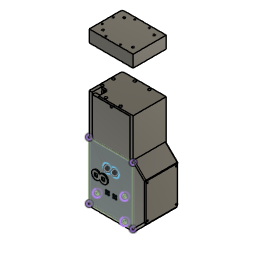
ExternalCardReaderHousingV3 v20 (Autodesk Fusion 360 design; units mm, degrees)
Autodesk Fusion 360 part; units mm, degrees
note: some values were not read from the file. Set by a fixed rule: which face or edge a step refers to.
(part 1 of 2)
sketch "ReaderBodyHalf" plane through (0, 0, 0) normal (0, 0, 1) x (1, 0, 0)
  line L0 (0, 0) -> (102, 0)
  line L1 (102, 0) -> (102, 38.5)
  line L2 (102, 38.5) -> (0, 38.5)
  line L3 (0, 38.5) -> (0, 0)
  line L4 (7, 7) -> (95, 7)
  line L5 (95, 7) -> (95, 38.5)
  line L6 (7, 38.5) -> (7, 7)
  circle A0 centre (90.5, 11.5) radius 1.75
  circle A1 centre (90.5, 11.5) radius 5.75
  circle A2 centre (11.5, 11.5) radius 1.75
  circle A3 centre (11.5, 11.5) radius 5.75
  line L7 (90.5, 17.25) -> (95, 17.25)
  line L8 (90.5, 11.5) -> (84.75, 11.5)
  line L9 (84.75, 7) -> (84.75, 11.5)
  line L10 (11.5, 17.25) -> (7, 17.25)
  line L11 (17.25, 11.5) -> (17.25, 7)
  line L12 (95, 17.25) -> (102, 17.25)
  line L13 (95, 7) -> (102, 7)
  circle A4 centre (34, 5) radius 2.35
  circle A5 centre (34, 5) radius 5
  circle A6 centre (34, 5) radius 5
  circle A7 centre (34, 5) radius 2.35
  circle A8 centre (68, 5) radius 5
  circle A9 centre (68, 5) radius 2.35
  circle A10 centre (5, 25.6667) radius 5
  circle A11 centre (5, 25.6667) radius 2.35
  circle A12 centre (90.5, 11.5) radius 0.7071
  circle A13 centre (68, 5) radius 1.75
  circle A14 centre (34, 5) radius 1.75
  circle A15 centre (5, 25.6667) radius 1.75
  circle A16 centre (5, 25.6667) radius 3
  circle A17 centre (34, 5) radius 3
  circle A18 centre (68, 5) radius 3
  line L14 (71, 5) -> (71, 7)
  line L15 (65, 5) -> (65, 7)
  line L16 (37, 5) -> (37, 7)
  line L17 (31, 5) -> (31, 7)
  line L18 (5, 22.6667) -> (7, 22.6667)
  line L19 (5, 28.6667) -> (7, 28.6667)
  dimension "d1" = 102
  dimension "d9" = 7
  dimension "d10" = 7
  dimension "d21" = 11.5
  dimension "d23" = 11.5
  dimension "d24" = 3.5
  dimension "d25" = 3.5
  dimension "d29" = 11.5
  dimension "d30" = 11.5
  dimension "d31" = 11.5
  dimension "d32" = 11.5
  dimension "d33" = 11.5
  dimension "d34" = 11.5
  dimension "d35" = 11.5
  dimension "d36" = 11.5
  dimension "d166" = 4.7
  dimension "d167" = 10
  dimension "d168" = 34
  dimension "d169" = 4.7
  dimension "d170" = 10
  dimension "d175" = 10
  dimension "d176" = 4.7
  dimension "d178" = 34
  dimension "d179" = 34
  dimension "d184" = 4.7
  dimension "d185" = 10
  dimension "d303" = 25.6667
  dimension "d340" = 38.5
  dimension "d392" = 3.5
  dimension "d393" = 3.5
  dimension "d394" = 3.5
  dimension "d470" = 6
  dimension "d471" = 6
  dimension "d472" = 6
  constraint horizontal L0
  constraint vertical L1
  constraint horizontal L2
  constraint vertical L3
  constraint coincident L0.start L3.end
  constraint horizontal L4
  constraint vertical L5
  constraint vertical L6
  constraint coincident A1 L7.start
  constraint tangent A1 L7
  constraint coincident L5 L7.end
  constraint perpendicular L5 L7
  constraint coincident A0.centre A1.centre
  constraint coincident A1 L8.end
  constraint parallel L4 L8
  constraint coincident L4 L9.start
  constraint tangent A1 L9
  constraint coincident A3 L10.start
  constraint coincident L6 L10.end
  constraint tangent A3 L10
  constraint perpendicular L6 L10
  constraint coincident A3 L11.start
  constraint coincident L4 L11.end
  constraint tangent A3 L11
  constraint perpendicular L4 L11
  constraint coincident L1 L12.end
  constraint perpendicular L1 L12
  constraint coincident L1 L13.end
  constraint perpendicular L1 L13
  constraint concentric A4 A5
  constraint concentric A6 A7
  constraint concentric A10 A11
  constraint coincident L2 L5.end
  constraint coincident L2 L6.start
  constraint concentric A1 A12
  constraint concentric A9 A13
  constraint concentric A5 A14
  constraint concentric A10 A15
  constraint concentric A10 A16
  constraint concentric A14 A17
  constraint concentric A13 A18
  constraint coincident A18 L14.start
  constraint coincident L4 L14.end
  constraint tangent A18 L14
  constraint perpendicular L4 L14
  constraint coincident A18 L15.start
  constraint coincident L4 L15.end
  constraint tangent A18 L15
  constraint perpendicular L4 L15
  constraint coincident A17 L16.start
  constraint coincident L4 L16.end
  constraint tangent A17 L16
  constraint perpendicular L4 L16
  constraint coincident A17 L17.start
  constraint coincident L4 L17.end
  constraint tangent A17 L17
  constraint perpendicular L4 L17
  constraint coincident A16 L18.start
  constraint coincident L6 L18.end
  constraint tangent A16 L18
  constraint perpendicular L6 L18
  constraint coincident A16 L19.start
  constraint coincident L6 L19.end
  constraint tangent A16 L19
  constraint perpendicular L6 L19
  measures "d1" distance of L0.start L0.end
  measures "d9" distance of L3 L6
  measures "d10" distance of L0 L4
  measures "d21" diameter of A3
  measures "d23" diameter of A1
  measures "d24" diameter of A0
  measures "d25" diameter of A2
  measures "d29" distance of L0 A0.centre
  measures "d30" distance of L1 A0.centre
  measures "d31" distance of L0 A2.centre
  measures "d32" distance of L3 A2.centre
  measures "d33" distance of L3 A2.centre
  measures "d34" distance of L0 A2.centre
  measures "d35" distance of L0 A0.centre
  measures "d36" distance of L1 A0.centre
  measures "d166" diameter of A4
  measures "d167" diameter of A5
  measures "d168" distance of L3 A4.centre
  measures "d169" diameter of A7
  measures "d170" diameter of A6
  measures "d175" diameter of A8
  measures "d176" diameter of A9
  measures "d178" distance of L1 A8.centre
  measures "d179" distance of L1 A8.centre
  measures "d184" diameter of A11
  measures "d185" diameter of A10
  measures "d303" distance of L0 A10.centre
  measures "d340" distance of L0.start L2.end
  measures "d392" diameter of A13
  measures "d393" diameter of A14
  measures "d394" diameter of A15
  measures "d470" diameter of A16
  measures "d471" diameter of A17
  measures "d472" diameter of A18
extrude "Extrude1" add sketch "ReaderBodyHalf" along normal blind 134 contours L0 L3 L4 L6 A3 A5 A6 A10 | L0 L4 A5 A6 A8 | L4 A5 A6 A17 L16 L17 | L2 L3 L6 A10 | L6 A10 A16 L18 L19 | L0 L1 L4 A1 L13 A8 | L4 A8 A18 L14 L15 | L4 A17 L17 | L6 A16 L19 | L6 A16 L18 | L4 A18 L15 | L4 A3 | L4 A4 A7 A17 | L4 A17 L16 | L6 A11 A16 | L6 A3 | L4 A9 A18 | L4 A18 L14 | L4 A4 A7 | L6 A11 | L4 A1 | L4 A9 | A13 | A14 | A15 picked at (31.228, 4.8338) picked at (4.8372, 28.4387) picked at (65.228, 4.8338) picked at (32.7196, 6.7212) picked at (2.8543, 25.6667) picked at (66.7196, 6.7212) makes body 1
extrude "Extrude2" add sketch "ReaderBodyHalf" along normal blind 6 contours L4 A3 L11 | L6 A3 L10 | L1 L5 A1 L12 L13 | L4 L6 A3 | L4 L5 A1 | L4 A1 L9 | L4 L6 A3 | L5 A1 L7 | L4 L5 A1 | L5 A1 bodies 1
extrude "Extrude16" add sketch "ReaderBodyHalf" against normal blind 8 from surface at 134 contours L4 A5 A6 A17 | L6 A10 A16 | L4 A8 A18 | L4 A4 A7 A17 | L6 A11 A16 | L4 A9 A18 | L4 A4 A7 | L6 A11 | L4 A9 picked at (32.6487, 7.4264) picked at (7.4264, 27.018) picked at (66.6487, 7.4264) picked at (34, 7.1167) picked at (7.0503, 25.3511) picked at (68.0958, 7.167) bodies 1
revolve "Revolve4" add 1 faces at (68.353, 8.1961, 126) angle 90 about axis through (63.4174, 7, 126) along (-1, 0, 0) on bodies 1 bodies 1
revolve "Revolve5" add 1 faces at (32.9452, 8.3501, 126) angle 90 about axis through (29.4174, 7, 126) along (-1, 0, 0) on bodies 1 bodies 1
revolve "Revolve6" add 1 faces at (8.3577, 25.1904, 126) angle 90 about axis through (7, 30.2492, 126) along (0, 1, 0) on bodies 1 bodies 1
extrude "Extrude17" cut sketch "ReaderBodyHalf" against normal blind 4 from surface at 134 contours L4 A4 A7 | L4 A4 A7 | L6 A11 | L6 A11 | L4 A9 | L4 A9 | A13 | A14 | A15 bodies 1
sketch "TopInsertHole alighment" plane through (102, 0, 0) normal (1, 0, 0) x (0, 1, 0)
  line L0 (0, 0) -> (17.25, 0)
  line L1 (17.25, 6) -> (7, 6)
  line L2 (0, 0) -> (77, 0)
  line L3 (77, 0) -> (77, 109.8006)
  line L4 (77, 109.8006) -> (0, 109.8006)
  line L5 (0, 109.8006) -> (0, 0)
  circle A0 centre (72, 28) radius 5
  circle A1 centre (72, 28) radius 2.35
  circle A2 centre (72, 104.8006) radius 2.35
  circle A3 centre (72, 104.8006) radius 5
  circle A4 centre (5, 104.8006) radius 2.35
  circle A5 centre (5, 104.8006) radius 5
  circle A6 centre (5, 28) radius 2.35
  circle A7 centre (5, 28) radius 5
  line L6 (64, 97.8006) -> (13, 97.8006)
  line L7 (13, 97.8006) -> (13, 33.8006)
  line L8 (13, 33.8006) -> (64, 33.8006)
  line L9 (64, 33.8006) -> (64, 97.8006)
  circle A8 centre (59.5, 89.0506) radius 2.35
  circle A9 centre (59.5, 43.0506) radius 2.35
  circle A10 centre (59.5, 89.0506) radius 5
  circle A11 centre (59.5, 43.0506) radius 5
  circle A12 centre (72, 28) radius 1.75
  circle A13 centre (72, 104.8006) radius 1.75
  circle A14 centre (5, 28) radius 1.75
  circle A15 centre (5, 104.8006) radius 1.75
  line L10 (17.25, 0) -> (17.25, 6)
  line L11 (0, 134) -> (0, 0)
  line L12 (7, 6) -> (7, 134)
  line L13 (7, 134) -> (0, 134)
  circle A16 centre (17.5, 89.0506) radius 5
  circle A17 centre (17.5, 89.0506) radius 2.35
  circle A18 centre (17.5, 43.0506) radius 5
  circle A19 centre (17.5, 43.0506) radius 2.35
  line L14 (77, 0) -> (77, -7)
  line L15 (77, -7) -> (0, -7)
  line L16 (0, -7) -> (0, 0)
  dimension "d218" = 10
  dimension "d219" = 5
  dimension "d221" = 4.7
  dimension "d222" = 4.7
  dimension "d223" = 4.7
  dimension "d224" = 4.7
  dimension "d225" = 10
  dimension "d226" = 10
  dimension "d227" = 10
  dimension "d231" = 5
  dimension "d232" = 5
  dimension "d233" = 5
  dimension "d280" = 64
  dimension "d281" = 51
  dimension "d282" = 13
  dimension "d283" = 12
  dimension "d284" = 4.7
  dimension "d285" = 4.7
  dimension "d286" = 4.5
  dimension "d287" = 4.5
  dimension "d288" = 8.75
  dimension "d289" = 46
  dimension "d290" = 10
  dimension "d291" = 10
  dimension "d295" = 3.5
  dimension "d296" = 3.5
  dimension "d297" = 3.5
  dimension "d298" = 3.5
  dimension "d346" = 4.7
  dimension "d347" = 4.7
  dimension "d348" = 46
  dimension "d349" = 10
  dimension "d350" = 10
  dimension "d351" = 4.5
  dimension "d352" = 4.5
  dimension "d353" = 7
  dimension "d354" = 35
  dimension "d355" = 35
  dimension "d357" = 5
  dimension "d358" = 5
  dimension "d359" = 8.75
  dimension "d360" = 13
  constraint horizontal L2
  constraint vertical L3
  constraint horizontal L4
  constraint vertical L5
  constraint coincident L0.start L2.start
  constraint concentric A0 A1
  constraint concentric A2 A3
  constraint concentric A4 A5
  constraint concentric A6 A7
  constraint horizontal L6
  constraint vertical L7
  constraint horizontal L8
  constraint vertical L9
  constraint concentric A8 A10
  constraint concentric A9 A11
  constraint concentric A0 A12
  constraint concentric A3 A13
  constraint concentric A7 A14
  constraint concentric A5 A15
  constraint concentric A16 A17
  constraint concentric A18 A19
  constraint perpendicular L2 L14
  constraint perpendicular L14 L15
  constraint perpendicular L2 L16
  measures "d218" diameter of A0
  measures "d219" distance of L3 A0.centre
  measures "d221" diameter of A1
  measures "d222" diameter of A6
  measures "d223" diameter of A4
  measures "d224" diameter of A2
  measures "d225" diameter of A7
  measures "d226" diameter of A5
  measures "d227" diameter of A3
  measures "d231" distance of L5 A6.centre
  measures "d232" distance of L5 A4.centre
  measures "d233" distance of L3 A2.centre
  measures "d280" distance of L6.end L7.end
  measures "d281" distance of L6.start L6.end
  measures "d282" distance of L3 L9
  measures "d283" distance of L4 L6
  measures "d284" diameter of A8
  measures "d285" diameter of A9
  measures "d286" distance of L9 A8.centre
  measures "d287" distance of L9 A9.centre
  measures "d288" distance of L6 A8.centre
  measures "d289" distance of A8.centre A9.centre
  measures "d290" diameter of A10
  measures "d291" diameter of A11
  measures "d295" diameter of A12
  measures "d296" diameter of A13
  measures "d297" diameter of A14
  measures "d298" diameter of A15
  measures "d346" diameter of A17
  measures "d347" diameter of A19
  measures "d348" distance of A16.centre A18.centre
  measures "d349" diameter of A16
  measures "d350" diameter of A18
  measures "d351" distance of L7 A16.centre
  measures "d352" distance of L7 A18.centre
  measures "d353" distance of L2.end L14.end
  measures "d354" distance of A0.centre L15
  measures "d355" distance of A6.centre L15
  measures "d357" distance of L4 A2.centre
  measures "d358" distance of L4 A4.centre
  measures "d359" distance of L6 A16.centre
  measures "d360" distance of L5 L7
extrude "Extrude18" add sketch "TopInsertHole alighment" against normal blind 8 contours A6 A7 L12 | A4 A5 L12 | A6 A7 L12 | A4 A5 L12 | A6 L12 | A6 L12 | A4 L12 | A4 L12 | A14 | A15 bodies 1
extrude "Extrude19" cut sketch "TopInsertHole alighment" against normal blind 4 contours A6 L12 | A6 L12 | A4 L12 | A4 L12 | A14 | A15 bodies 1
extrude "Extrude29" cut sketch "TopInsertHole alighment" against normal blind 3 from surface at -4 contours A14 | A15 bodies 1
mirror "Mirror1" about plane through (7, 38.5, 0) normal (0, 1, 0) of bodies 1 makes body 2
sketch "PingulpMount" plane through (0, 0, 0) normal (0, 1, 0) x (1, 0, 0)
  line L0 (0, -1.75) -> (0, -22.5)
  circle A0 centre (18.5001, -30.5) radius 2.5
  circle A1 centre (82.5001, -5) radius 4.25
  line L1 (89.0001, 6) -> (89.0001, -68)
  line L2 (0.0001, -68) -> (0.0001, 6)
  circle A2 centre (18.5001, -30.5) radius 4.25
  circle A3 centre (82.5001, -56) radius 4.25
  circle A4 centre (82.5001, -5) radius 2.5
  line L3 (0.0001, 6) -> (89.0001, 6)
  circle A5 centre (82.5001, -56) radius 2.5
  line L4 (89.0001, -68) -> (0.0001, -68)
  point P0 (5, 0)
  dimension "d324" = 74
  dimension "d325" = 89
  dimension "d326" = 0.0001
  dimension "d327" = 5
  dimension "d328" = 5
  dimension "d329" = 5
  dimension "d330" = 6.5
  dimension "d331" = 11
  dimension "d332" = 6.5
  dimension "d333" = 51
  dimension "d334" = 36.5
  dimension "d335" = 70.5
  dimension "d336" = 8.5
  dimension "d337" = 8.5
  dimension "d338" = 8.5
  constraint horizontal L3
  constraint vertical L1
  constraint horizontal L4
  constraint vertical L2
  constraint concentric A0 A2
  constraint concentric A3 A5
  constraint concentric A1 A4
  measures "d324" distance of L2.end L2.start
  measures "d325" distance of L1.start L2.end
  measures "d326" distance of L0 L2
  measures "d327" diameter of A0
  measures "d328" diameter of A5
  measures "d329" diameter of A4
  measures "d330" distance of A1.centre L1
  measures "d331" distance of A1.centre L3
  measures "d332" distance of A3.centre L1
  measures "d333" distance of A3.centre A1.centre
  measures "d334" distance of A0.centre L3
  measures "d335" distance of A0.centre L1
  measures "d336" diameter of A2
  measures "d337" diameter of A3
  measures "d338" diameter of A1
extrude "Extrude12" cut sketch "PingulpMount" against normal blind 2 from surface at 7 contours A0 | A1 | A2 | A3 | A4 | A5 bodies 1
extrude "Extrude11" cut sketch "PingulpMount" along normal blind 10 contours A0 | A4 | A5 bodies 1
sketch "PiMount" plane through (0, 70, 0) normal (0, -1, 0) x (1, 0, 0)
  line L0 (102, 100.218) -> (94, 100.218)
  line L1 (94, 100.218) -> (94, 109.3832)
  line L2 (94, 109.3832) -> (102, 109.3832)
  line L3 (102, 109.3832) -> (102, 134)
  line L4 (102, 134) -> (72.5826, 134)
  line L5 (7, 134) -> (7, 6)
  line L6 (7, 6) -> (17.25, 6)
  line L7 (17.25, 6) -> (17.25, 0)
  line L8 (17.25, 0) -> (84.75, 0)
  line L9 (84.75, 0) -> (84.75, 6)
  line L10 (84.75, 6) -> (102, 6)
  line L11 (102, 6) -> (102, 23.4174)
  line L12 (102, 23.4174) -> (94, 23.4174)
  line L13 (94, 23.4174) -> (94, 32.5826)
  line L14 (94, 32.5826) -> (102, 32.5826)
  line L15 (102, 32.5826) -> (102, 100.218)
  circle A0 centre (15.5869, 30.5277) radius 1
  circle A1 centre (64.5844, 31.0206) radius 1
  circle A2 centre (15, 88.5248) radius 1
  circle A3 centre (63.9975, 89.0206) radius 1
  circle A4 centre (15, 88.5248) radius 3
  circle A5 centre (15.5869, 30.5277) radius 3
  circle A6 centre (64.5844, 31.0206) radius 3
  circle A7 centre (63.9975, 89.0206) radius 3
  line L16 (72.5826, 134) -> (72.5826, 126)
  arc A8 (63.4174, 126) -> (72.5826, 126) centre (68, 128) ccw
  line L17 (63.4174, 126) -> (63.4174, 134)
  line L18 (63.4174, 134) -> (38.5826, 134)
  line L19 (38.5826, 134) -> (38.5826, 126)
  arc A9 (29.4174, 126) -> (38.5826, 126) centre (34, 128) ccw
  line L20 (29.4174, 126) -> (29.4174, 134)
  line L21 (29.4174, 134) -> (7, 134)
  dimension "d306" = 49
  dimension "d307" = 49
  dimension "d308" = 58
  dimension "d309" = 2
  dimension "d310" = 2
  dimension "d311" = 2
  dimension "d312" = 2
  dimension "d313" = 6
  dimension "d314" = 6
  dimension "d315" = 6
  dimension "d316" = 6
  dimension "d317" = 8
  dimension "d318" = 58
  constraint concentric A2 A4
  constraint concentric A0 A5
  constraint concentric A1 A6
  constraint concentric A3 A7
  measures "d306" distance of A0.centre A1.centre
  measures "d307" distance of A2.centre A3.centre
  measures "d308" distance of A0.centre A2.centre
  measures "d309" diameter of A2
  measures "d310" diameter of A3
  measures "d311" diameter of A0
  measures "d312" diameter of A1
  measures "d313" diameter of A4
  measures "d314" diameter of A7
  measures "d315" diameter of A5
  measures "d316" diameter of A6
  measures "d317" distance of L5 A2.centre
  measures "d318" vertical distance of A1.centre A3.centre
extrude "Extrude27" add sketch "PiMount" along normal blind 5 contours A4 | A5 | A6 | A7 bodies 2
extrude "Extrude28" cut sketch "PiMount" against normal blind 4 contours A0 | A1 | A2 | A3 bodies 2
fillet "Fillet8" radius 4.5 1 edges at (0, 77, 67) on bodies 2
sketch "LcdHousing" plane through (0, 0, 0) normal (0, 1, 0) x (1, 0, 0)
  line L0 (102, 7) -> (130.2828, -21.2858)
  line L1 (130.2828, -21.2858) -> (130.2828, -110)
  line L2 (102, -110) -> (102, 7)
  line L3 (102, -110) -> (102, -138)
  line L4 (102, -138) -> (130.2828, -110)
  dimension "d236" = 40
  dimension "d383" = 28
  measures "d236" distance of L0.start L0.end
  measures "d383" distance of L2.start L3.end
extrude "Extrude20" add sketch "LcdHousing" along normal blind 77 separate body makes body 3
shell "Shell1" thickness 4 removed faces 2 at (102, 25.6667, 71) at (102, 25.6667, 119.3333) on bodies 3
extrude "Extrude24" add sketch "TopInsertHole alighment" along normal blind 25 contours A0 | A6 A7 L12 | A4 A5 L12 | A6 A7 L12 | A4 A5 L12 | A6 L12 | A6 L12 | A3 | A4 L12 | A4 L12 | A1 | A2 bodies 3
extrude "Extrude25" cut sketch "TopInsertHole alighment" along normal blind 29 contours A12 | A13 | A14 | A15 bodies 3
sketch "LcdFace" plane through (54.5054, 0, -54.4996) normal (0.707145, 0, -0.707069) x (0, 1, 0)
  line L0 (0, 107.171) -> (0, 67.171)
  line L1 (77, 67.171) -> (77, 107.171)
  line L2 (13, 79.171) -> (64, 79.171)
  line L3 (64, 79.171) -> (64, 99.171)
  line L4 (64, 99.171) -> (13, 99.171)
  line L5 (13, 99.171) -> (13, 79.171)
  line L6 (64, 75.671) -> (13, 75.671)
  line L7 (13, 75.671) -> (13, 102.671)
  line L8 (13, 102.671) -> (64, 102.671)
  line L9 (64, 102.671) -> (64, 75.671)
  circle A0 centre (60.25, 100.671) radius 1
  circle A1 centre (16.75, 100.671) radius 1
  circle A2 centre (17, 77.671) radius 1
  circle A3 centre (60.5, 77.671) radius 1
  line L10 (29, 102.671) -> (29, 99.171)
  line L11 (48, 102.671) -> (48, 99.171)
  line L12 (77, 107.171) -> (0, 107.171)
  line L13 (0, 67.171) -> (77, 67.171)
  dimension "d244" = 51
  dimension "d245" = 20
  dimension "d246" = 13
  dimension "d252" = 51
  dimension "d253" = 27
  dimension "d254" = 3.5
  dimension "d255" = 13
  dimension "d262" = 2
  dimension "d263" = 3.75
  dimension "d264" = 2
  dimension "d265" = 2
  dimension "d266" = 2
  dimension "d267" = 2
  dimension "d268" = 43.5
  dimension "d269" = 23
  dimension "d270" = 43.5
  dimension "d271" = 23
  dimension "d272" = 2
  dimension "d299" = 16
  dimension "d300" = 16
  constraint horizontal L2
  constraint vertical L3
  constraint horizontal L4
  constraint vertical L5
  constraint horizontal L6
  constraint vertical L7
  constraint horizontal L8
  constraint vertical L9
  constraint coincident L8 L10.start
  constraint coincident L4 L10.end
  constraint perpendicular L4 L10
  constraint coincident L8 L11.start
  constraint coincident L4 L11.end
  constraint perpendicular L4 L11
  measures "d244" distance of L3.end L4.end
  measures "d245" distance of L2.end L3.end
  measures "d246" distance of L0 L5
  measures "d252" distance of L6.start L6.end
  measures "d253" distance of L6.start L8.end
  measures "d254" distance of L2 L6
  measures "d255" distance of L0 L7
  measures "d262" diameter of A0
  measures "d263" distance of L9 A0.centre
  measures "d264" distance of L8 A0.centre
  measures "d265" diameter of A1
  measures "d266" diameter of A2
  measures "d267" diameter of A3
  measures "d268" horizontal distance of A0.centre A1.centre
  measures "d269" vertical distance of A1.centre A2.centre
  measures "d270" horizontal distance of A2.centre A3.centre
  measures "d271" vertical distance of A0.centre A3.centre
  measures "d272" distance of L8 A1.centre
  measures "d299" distance of L7 L10
  measures "d300" distance of L9 L11
extrude "Extrude21" cut sketch "LcdFace" against normal blind 8 contours L2 L3 L4 L5 L7 L9 bodies 3
extrude "Extrude22" add sketch "LcdFace" against normal blind 8 contours L2 L6 L7 L9 | L4 L7 L8 L10 | L4 L8 L9 L11 | L4 L8 L10 L11 | A0 | A1 | A2 | A3 bodies 3
extrude "Extrude23" cut sketch "LcdFace" along normal blind 4 from surface at -8 contours L4 L8 L10 L11 | A0 | A1 | A2 | A3 bodies 3
extrude "Extrude26" add sketch "TopInsertHole alighment" against normal blind 4 from surface at 24.2828 contours L9 A10 | L9 A10 | L7 A16 | L7 A16 | L9 A11 | L9 A11 | L7 A18 | L7 A18 bodies 3
sketch "Sketch10" plane through (0, 0, 0) normal (0, 0, 1) x (1, 0, 0)
  line L0 (102, 77) -> (0, 77)
  line L1 (0, 77) -> (0, 0)
  line L2 (0, 0) -> (102, 0)
  line L3 (102, 0) -> (102, 77)
  constraint horizontal L0
  constraint vertical L1
  constraint horizontal L2
  constraint vertical L3
  constraint coincident L1.end L2.start
extrude "Extrude30" add sketch "Sketch10" against normal blind 7 separate body makes body 4
fillet "Fillet9" radius 4.5 4 edges at (0, 0, -3.5) (102, 0, -3.5) (102, 77, -3.5) (0, 77, -3.5) on bodies 4
chamfer "Chamfer1" distance 2 distance2 7 8 edges at (51, 77, -7) (100.682, 75.682, -7) (102, 38.5, -7) (100.682, 1.318, -7) (51, 0, -7) (1.318, 1.318, -7) (0, 38.5, -7) (1.318, 75.682, -7) measured on face at (66.5, 25.6667, -7) measured on face at (99.562, 76.4998, -2.3333) measured on face at (66.5, 25.6667, -7) measured on face at (99.562, 0.5002, -2.3333) measured on face at (66.5, 25.6667, -7) measured on face at (0.0204, 4.0722, -2.3333) measured on face at (66.5, 25.6667, -7) measured on face at (0.9628, 75.2817, -2.3333) on bodies 4
sketch "Sketch11" plane through (102, 0, 0) normal (-1, 0, 0) x (0, -1, 0)
  arc A0 (-73, 106.2368) -> (-73, 103.3645) centre (-72, 104.8006) ccw
  arc A1 (-4, 103.3645) -> (-4, 106.2368) centre (-5, 104.8006) ccw
  line L0 (-4, 103.3645) -> (-4, 99.9016)
  line L1 (-4, 110) -> (-4, 109.6996)
  line L2 (-4, 32.899) -> (-4, 29.4361)
  arc A2 (-4, 26.5639) -> (-4, 29.4361) centre (-5, 28) ccw
  line L3 (-4, 26.5639) -> (-4, 23.101)
  line L4 (-4, 23.101) -> (-4, -1.3428)
  line L5 (-4, -1.3428) -> (-73, -1.3428)
  line L6 (-73, 109.6996) -> (-73, 110)
  line L7 (-73, 23.101) -> (-73, 26.5639)
  arc A3 (-73, 29.4361) -> (-73, 26.5639) centre (-72, 28) ccw
  line L8 (-73, 29.4361) -> (-73, 32.899)
  line L9 (-73, 32.899) -> (-73, 99.9016)
  line L10 (-73, 99.9016) -> (-73, 103.3645)
  line L11 (0, -7) -> (0, 110)
  line L12 (-77, 110) -> (-77, -7)
  line L13 (-77, -7) -> (0, -7)
  line L14 (0, -7) -> (-77, -7)
  line L15 (-77, -7) -> (-77, 0)
  line L16 (-77, 0) -> (0, 0)
  line L17 (0, 0) -> (0, -7)
  line L18 (-73, 106.2368) -> (-73, 109.6996)
  line L19 (-73, 110) -> (-77, 110)
  line L20 (0, 110) -> (-4, 110)
  line L21 (-4, 109.6996) -> (-4, 106.2368)
  line L22 (-4, 99.9016) -> (-4, 32.899)
  line L23 (-73, -1.3428) -> (-73, 23.101)
  constraint horizontal L14
  constraint vertical L15
  constraint horizontal L16
  constraint vertical L17
  constraint coincident L11.start L13.end
extrude "Extrude31" add sketch "Sketch11" along normal blind 5 separate body contours L4 L5 L11 L12 L13 L14 L15 L16 L17 L23 | L4 L5 L16 L23 makes body 5
chamfer "Chamfer4" distance 2 distance2 7 1 edges at (99.5, 0, -7) measured on face at (100.3333, 51.3333, -7) on bodies 5
chamfer "Chamfer4" distance 7 distance2 2 1 edges at (99.5, 77, -7) measured on face at (100.3333, 77, -2.3333) on bodies 5
chamfer "Chamfer2" distance 5 distance2 2 1 edges at (116.1414, 0, 7.1429) measured on face at (116.1414, 0, 65.5) on bodies 3
chamfer "Chamfer2" distance 5 distance2 2 1 edges at (116.1414, 77, 7.1429) measured on face at (110.3333, 77, 53.6002) on bodies 3
combine "Combine2" operation cut target body 5 tool bodies 4 keep tools
combine "Combine3" operation add target body 5 tool bodies 3
fillet "Fillet12" radius 2 8 edges at (116.1414, 0, 124) (116.1414, 77, 124) (130.2828, 0, 69.1786) (130.2828, 77, 69.1786) (130.2828, 1, 24.8215) (130.2828, 38.5, 21.2858) (130.2828, 76, 24.8215) (130.2828, 38.5, 110) on bodies 5
extrude "Extrude32" add sketch "ReaderBodyHalf" along normal blind 28 from surface at 134 separate body contours L0 L3 L4 L6 A3 A5 A6 A10 | L0 L4 A5 A6 A8 | L4 A5 A6 A17 L16 L17 | L2 L3 L6 A10 | L6 A10 A16 L18 L19 | L0 L1 L4 A1 L13 A8 | L4 A8 A18 L14 L15 | L4 A5 A6 A17 | L2 L4 L5 L6 A1 A3 L7 L9 L10 L11 A5 A6 A8 A10 | L6 A10 A16 | L4 A8 A18 | L4 A3 L11 | L4 A17 L17 | L6 A16 L19 | L6 A16 L18 | L6 A3 L10 | L1 L5 A1 L12 L13 | L4 A18 L15 | L4 A3 | L4 L6 A3 | L4 A4 A7 A17 | L4 A4 A7 A17 | L4 A17 L16 | L1 L2 L5 L12 | L6 A11 A16 | L6 A11 A16 | L6 A3 | L4 L5 A1 | L4 A9 A18 | L4 A9 A18 | L4 A18 L14 | L4 A1 L9 | L4 L6 A3 | L4 A4 A7 | L4 A4 A7 | L5 A1 L7 | L6 A11 | L6 A11 | L4 A1 | L4 L5 A1 | L5 A1 | L4 A9 | L4 A9 | A0 | A2 | A12 | A13 | A14 | A15 makes body 6
extrude "Extrude33" cut sketch "ReaderBodyHalf" along normal blind 28 from surface at 134 contours A13 | A14 | A15 bodies 6
mirror "Mirror2" about plane through (7, 38.5, 134) normal (0, 1, 0) of bodies 6 merged
fillet "Fillet11" radius 4.5 1 edges at (0, 77, 148) on bodies 6
shell "Shell2" thickness 4 removed faces 1 at (91.0304, 27.7894, 134) on bodies 6
sketch "Sketch12" plane through (0, 0, 0) normal (-1, 0, 0) x (0, -1, 0)
  line L0 (-72.5, 162) -> (-72.5, 134)
  line L1 (-72.5, 134) -> (0, 134)
  line L2 (0, 134) -> (0, 162)
  line L3 (0, 162) -> (-72.5, 162)
  line L4 (-72.0657, 134) -> (-57.0657, 134)
  arc A0 (-57.0657, 134) -> (-72.0657, 134) centre (-64.5657, 134.0205) ccw
  line L5 (-20.0657, 134) -> (-5.0657, 134)
  arc A1 (-5.0657, 134) -> (-20.0657, 134) centre (-12.5657, 134.0141) ccw
  dimension "d409" = 15
  dimension "d412" = 15
  constraint coincident L1 L4.start
  constraint coincident L1 L4.end
  constraint perpendicular L0 L4
  measures "d409" distance of L4.start L4.end
  measures "d412" distance of L5.start L5.end
extrude "Extrude35" cut sketch "Sketch12" against normal blind 9 contours L1 L4 A0 | L1 L5 A1 bodies 6
sketch "ReleayBoardMount" plane through (0, 0, 162) normal (0, 0, 1) x (-1, 0, 0)
  arc A0 (-4.5, -77) -> (0, -72.5) centre (-4.5, -72.5) ccw
  line L0 (0, -72.5) -> (0, 0)
  line L1 (0, 0) -> (-102, 0)
  line L2 (-102, 0) -> (-102, -77)
  line L3 (-102, -77) -> (-4.5, -77)
  circle A1 centre (-5, -25.6667) radius 1.75
  circle A2 centre (-34, -5) radius 1.75
  circle A3 centre (-68, -5) radius 1.75
  circle A4 centre (-68, -72) radius 1.75
  circle A5 centre (-34, -72) radius 1.75
  circle A6 centre (-5, -51.3333) radius 1.75
  circle A7 centre (-18, -63.4) radius 2.35
  circle A8 centre (-87.6, -63.4) radius 2.35
  circle A9 centre (-18, -14) radius 2.35
  circle A10 centre (-87.6, -14) radius 2.35
  circle A11 centre (-18, -63.4) radius 4.7
  circle A12 centre (-18, -14) radius 4.7
  circle A13 centre (-87.6, -63.4) radius 4.7
  circle A14 centre (-87.6, -14) radius 4.7
  point P0 (0, -12.5657)
  dimension "d415" = 69.6
  dimension "d416" = 69.6
  dimension "d417" = 49.4
  dimension "d418" = 49.4
  dimension "d419" = 4.7
  dimension "d420" = 4.7
  dimension "d421" = 4.7
  dimension "d422" = 4.7
  dimension "d423" = 18
  dimension "d424" = 14
  dimension "d425" = 9.4
  dimension "d426" = 9.4
  dimension "d427" = 9.4
  dimension "d428" = 9.4
  constraint concentric A7 A11
  constraint concentric A9 A12
  constraint concentric A8 A13
  constraint concentric A10 A14
  measures "d415" distance of A7.centre A8.centre
  measures "d416" distance of A9.centre A10.centre
  measures "d417" distance of A7.centre A9.centre
  measures "d418" distance of A8.centre A10.centre
  measures "d419" diameter of A7
  measures "d420" diameter of A8
  measures "d421" diameter of A9
  measures "d422" diameter of A10
  measures "d423" horizontal distance of A9.centre P0
  measures "d424" distance of L1 A9.centre
  measures "d425" diameter of A11
  measures "d426" diameter of A13
  measures "d427" diameter of A14
  measures "d428" diameter of A12
extrude "Extrude36" cut sketch "ReleayBoardMount" against normal blind 5 contours A7 | A8 | A9 | A10 bodies 6
extrude "Extrude37" add sketch "ReleayBoardMount" against normal blind 4 contours A11 | A12 | A13 | A14 bodies 6
move_body "Move3" bodies 6 to x (1, 0, 0) y (0, 1, 0) z (0, 0, 1) at (0, 0, 190)
extrude "Extrude38" add sketch "ReaderBodyHalf" along normal blind 94 from surface at 134 separate body contours L0 L3 L4 L6 A3 A5 A6 A10 | L0 L4 A5 A6 A8 | L4 A5 A6 A17 L16 L17 | L2 L3 L6 A10 | L6 A10 A16 L18 L19 | L0 L1 L4 A1 L13 A8 | L4 A8 A18 L14 L15 | L1 L5 A1 L12 L13 | L4 A3 | L1 L2 L5 L12 | L6 A3 | L4 A1 | L5 A1 makes body 7
extrude "Extrude39" add sketch "ReaderBodyHalf" along normal blind 7 from surface at 134 contours L4 A5 A6 A17 | L6 A10 A16 | L4 A8 A18 | L4 A17 L17 | L6 A16 L19 | L6 A16 L18 | L4 A18 L15 | L4 A4 A7 A17 | L4 A4 A7 A17 | L4 A17 L16 | L6 A11 A16 | L6 A11 A16 | L4 A9 A18 | L4 A9 A18 | L4 A18 L14 | L4 A4 A7 | L4 A4 A7 | L6 A11 | L6 A11 | L4 A9 | L4 A9 bodies 7
extrude "Extrude40" add sketch "ReaderBodyHalf" against normal blind 4 from surface at 228 contours L4 A5 A6 A17 | L2 L4 L5 L6 A1 A3 L7 L9 L10 L11 A5 A6 A8 A10 | L6 A10 A16 | L4 A8 A18 | L4 A3 L11 | L4 A17 L17 | L6 A16 L19 | L6 A16 L18 | L6 A3 L10 | L4 A18 L15 | L4 A3 | L4 L6 A3 | L4 A17 L16 | L6 A3 | L4 L5 A1 | L4 A18 L14 | L4 A1 L9 | L4 L6 A3 | L5 A1 L7 | L4 L5 A1 | A0 | A2 | A12 bodies 7
mirror "Mirror3" about plane through (7, 38.5, 134) normal (0, 1, 0) of bodies 7 merged
sketch "RelayBoxCrossSection" plane through (0, 0, 0) normal (0, -1, 0) x (1, 0, 0)
  line L0 (102, 134) -> (102, 228)
  line L1 (102, 228) -> (0, 228)
  line L2 (0, 228) -> (0, 134)
  line L3 (102, 228) -> (0, 228)
  circle A0 centre (26.5, 144) radius 2.35
  circle A1 centre (26.5, 213.6) radius 2.35
  circle A2 centre (75.9, 213.6) radius 2.35
  circle A3 centre (75.9, 144) radius 2.35
  circle A4 centre (75.9, 213.6) radius 4.7
  circle A5 centre (26.5, 213.6) radius 4.7
  circle A6 centre (26.5, 144) radius 4.7
  circle A7 centre (75.9, 144) radius 4.7
  line L4 (102, 228) -> (0, 228)
  line L5 (0, 228) -> (0, 134)
  line L6 (0, 134) -> (102, 134)
  line L7 (102, 134) -> (102, 228)
  line L8 (7, 134) -> (7, 228)
  line L9 (95, 134) -> (95, 228)
  line L10 (0, 224) -> (102, 224)
  line L11 (7, 139.0272) -> (12, 139.0272)
  line L12 (12, 139.0272) -> (12, 134)
  line L13 (89.9369, 134) -> (89.9369, 139.0272)
  line L14 (89.9369, 139.0272) -> (95, 139.0272)
  circle A8 centre (51.2, 220.6) radius 4.7
  circle A9 centre (51.2, 220.6) radius 2.35
  line L15 (46.5, 220.6) -> (46.5, 224)
  line L16 (55.9, 220.6) -> (55.9, 224)
  line L17 (7.25, 223.75) -> (94.75, 223.75)
  line L18 (94.75, 223.75) -> (94.75, 134.25)
  line L19 (94.75, 134.25) -> (7.25, 134.25)
  line L20 (7.25, 134.25) -> (7.25, 223.75)
  line L21 (40, 132) -> (61, 132)
  line L22 (61, 132) -> (61, 136)
  line L23 (61, 136) -> (40, 136)
  line L24 (40, 136) -> (40, 132)
  circle A10 centre (51.2, 220.6) radius 1.75
  dimension "d448" = 69.6
  dimension "d449" = 69.6
  dimension "d450" = 49.4
  dimension "d452" = 4.7
  dimension "d453" = 4.7
  dimension "d454" = 4.7
  dimension "d455" = 4.7
  dimension "d456" = 9.4
  dimension "d457" = 9.4
  dimension "d458" = 9.4
  dimension "d459" = 9.4
  dimension "d473" = 26.5
  dimension "d474" = 10
  dimension "d475" = 10
  dimension "d476" = 26.5
  dimension "d477" = 49.4
  dimension "d479" = 7
  dimension "d480" = 7
  dimension "d481" = 4
  dimension "d494" = 4.7
  dimension "d495" = 9.4
  dimension "d496" = 51.2
  dimension "d515" = 0.25
  dimension "d516" = 0.25
  dimension "d517" = 0.25
  dimension "d518" = 0.25
  dimension "d524" = 3.5
  constraint horizontal L3
  constraint coincident L0.end L1.start
  constraint concentric A2 A4
  constraint concentric A1 A5
  constraint concentric A0 A6
  constraint concentric A3 A7
  constraint horizontal L4
  constraint vertical L5
  constraint horizontal L6
  constraint vertical L7
  constraint coincident L2.end L5.end
  constraint coincident L6 L8.start
  constraint coincident L4 L8.end
  constraint perpendicular L4 L8
  constraint coincident L6 L9.start
  constraint coincident L4 L9.end
  constraint perpendicular L4 L9
  constraint coincident L5 L10.start
  constraint coincident L7 L10.end
  constraint perpendicular L7 L10
  constraint coincident L8 L11.start
  constraint perpendicular L8 L11
  constraint coincident L6 L12.end
  constraint perpendicular L6 L12
  constraint coincident L6 L13.start
  constraint perpendicular L6 L13
  constraint coincident L9 L14.end
  constraint perpendicular L9 L14
  constraint concentric A8 A9
  constraint coincident A8 L15.start
  constraint coincident L10 L15.end
  constraint tangent A8 L15
  constraint perpendicular L10 L15
  constraint coincident A8 L16.start
  constraint coincident L10 L16.end
  constraint tangent A8 L16
  constraint perpendicular L10 L16
  constraint horizontal L17
  constraint vertical L18
  constraint horizontal L19
  constraint vertical L20
  constraint horizontal L21
  constraint vertical L22
  constraint horizontal L23
  constraint vertical L24
  constraint concentric A9 A10
  measures "d448" distance of A0.centre A1.centre
  measures "d449" distance of A2.centre A3.centre
  measures "d450" distance of A0.centre A3.centre
  measures "d452" diameter of A2
  measures "d453" diameter of A1
  measures "d454" diameter of A0
  measures "d455" diameter of A3
  measures "d456" diameter of A5
  measures "d457" diameter of A4
  measures "d458" diameter of A6
  measures "d459" diameter of A7
  measures "d473" distance of A0.centre L5
  measures "d474" distance of A0.centre L6
  measures "d475" distance of A3.centre L6
  measures "d476" distance of A1.centre L5
  measures "d477" distance of A2.centre A1.centre
  measures "d479" distance of L7 L9
  measures "d480" distance of L5 L8
  measures "d481" distance of L4 L10
  measures "d494" diameter of A9
  measures "d495" diameter of A8
  measures "d496" distance of L5 A8.centre
  measures "d515" distance of L8 L20
  measures "d516" distance of L10 L17
  measures "d517" distance of L9 L18
  measures "d518" distance of L6 L19
  measures "d524" diameter of A10
extrude "Extrude41" cut sketch "RelayBoxCrossSection" against normal blind 12 contours L6 L9 L13 L14 L18 L19 | L9 L10 L14 L16 L17 L18 | L6 L13 L19 L22 | L10 A8 L16 L17 | L6 L19 L22 L24 | L11 L12 L13 L14 A8 L15 L16 L17 L18 L19 L20 L22 L23 L24 | L13 L14 L18 L19 | L10 A8 L17 | A8 L16 L17 | L6 L12 L19 L24 | L19 L22 L23 L24 | L8 L10 L11 L15 L17 L20 | L10 A8 L15 L17 | A8 L17 | L6 L8 L11 L12 L19 L20 | A8 L15 L17 | L11 L12 L19 L20 | A0 | A1 | A2 | A3 | A4 | A5 | A6 | A7 | A9 | A10 bodies 7
extrude "Extrude42" add sketch "RelayBoxCrossSection" along normal blind 4 from surface at -70 contours A4 | A5 | A6 | A7 bodies 7
fillet "Fillet13" radius 4.5 1 edges at (0, 77, 181) on bodies 7
sketch "CableOut" plane through (0, 0, 224) normal (0, 0, -1) x (1, 0, 0)
  line L0 (7, 0) -> (7, -22.6667)
  arc A0 (5, -28.6667) -> (5, -22.6667) centre (5, -25.6667) ccw
  line L1 (7, -54.3333) -> (7, -70)
  arc A1 (5, -54.3333) -> (5, -48.3333) centre (5, -51.3333) ccw
  line L2 (7, -70) -> (31, -70)
  arc A2 (37, -72) -> (31, -72) centre (34, -72) ccw
  arc A3 (71, -72) -> (65, -72) centre (68, -72) ccw
  line L3 (95, -70) -> (95, 0)
  line L4 (95, 0) -> (7, 0)
  line L5 (7, 0) -> (7, -22)
  line L6 (7, 0) -> (22, 0)
  line L7 (22, 0) -> (22, -17)
  line L8 (7, -22) -> (17, -22)
  arc A4 (17, -22) -> (22, -17) centre (17, -17) ccw
  circle A5 centre (34, -5) radius 3
  line L9 (7, -22.6667) -> (5, -22.6667)
  line L10 (5, -28.6667) -> (7, -28.6667)
  line L11 (7, -28.6667) -> (7, -48.3333)
  line L12 (7, -48.3333) -> (5, -48.3333)
  line L13 (5, -54.3333) -> (7, -54.3333)
  line L14 (31, -70) -> (31, -72)
  line L15 (37, -72) -> (37, -70)
  line L16 (37, -70) -> (65, -70)
  line L17 (65, -70) -> (65, -72)
  line L18 (71, -72) -> (71, -70)
  line L19 (71, -70) -> (95, -70)
  circle A6 centre (68, -5) radius 3
  dimension "d492" = 22
  dimension "d493" = 17
  constraint coincident L0.start L4.end
  constraint coincident L0 L5.end
  constraint perpendicular L4 L5
  constraint coincident L4 L6.end
  constraint perpendicular L4 L7
  constraint perpendicular L0 L8
  constraint tangent L7 A4
  constraint tangent L8 A4
  measures "d492" distance of L0.start L5.end
  measures "d493" distance of L6.end L7.end
extrude "Extrude47" add sketch "RelayBoxCrossSection" against normal blind 4 from surface at -7 contours L10 A8 L16 L17 | L10 A8 L17 | A8 L16 L17 | L10 A8 L15 L17 | A8 L17 | A8 L15 L17 bodies 7
revolve "Revolve8" add 1 faces at (47.3609, 11, 221.9899) angle 90 about axis through (55.9, 11, 224) along (1, 0, 0) on bodies 7 bodies 7
extrude "Extrude48" add sketch "RelayBoxCrossSection" against normal blind 1 from surface at -7 contours L6 L9 L13 L14 L18 L19 | L13 L14 L18 L19 | L6 L8 L11 L12 L19 L20 | L11 L12 L19 L20 bodies 7
revolve "Revolve9" add 1 faces at (10.3333, 8, 135.6757) angle 90 about axis through (7, 8, 139.0272) along (0, 0, 1) on bodies 7 bodies 7
revolve "Revolve10" add 1 faces at (93.3123, 8, 137.3515) angle 90 about axis through (95, 8, 134) along (0, 0, -1) on bodies 7 bodies 7
extrude "Extrude43" cut sketch "CableOut" against normal blind 10 contours L0 L4 L5 L6 L7 L8 A4 bodies 7
sketch "Sketch18" plane through (0, 0, 0) normal (-1, 0, 0) x (0, -1, 0)
  line L0 (-72.5, 228) -> (-72.5, 134)
  line L1 (-72.5, 134) -> (0, 134)
  line L2 (0, 134) -> (0, 228)
  line L3 (0, 228) -> (-72.5, 228)
  line L4 (-22, 220) -> (-27, 220)
  line L5 (-27, 220) -> (-27, 210)
  line L6 (-27, 210) -> (-22, 210)
  line L7 (-22, 210) -> (-22, 220)
  line L8 (-7, 220) -> (-12, 220)
  line L9 (-12, 220) -> (-12, 210)
  line L10 (-12, 210) -> (-7, 210)
  line L11 (-7, 210) -> (-7, 220)
  constraint horizontal L4
  constraint vertical L5
  constraint horizontal L6
  constraint vertical L7
  constraint horizontal L8
  constraint vertical L9
  constraint horizontal L10
  constraint vertical L11
extrude "Extrude45" cut sketch "Sketch18" against normal blind 8 contours L4 L5 L6 L7 | L8 L9 L10 L11 bodies 7
extrude "Extrude46" add sketch "RelayBoxCrossSection" against normal blind 7 separate body contours L11 L12 L13 L14 A8 L15 L16 L17 L18 L19 L20 L22 L23 L24 | L13 L14 L18 L19 | A8 L16 L17 | L19 L22 L23 L24 | A8 L17 | A8 L15 L17 | L11 L12 L19 L20 | A0 | A1 | A2 | A3 | A4 | A5 | A6 | A7 | A9 makes body 8
extrude "Extrude49" cut sketch "ReaderBodyHalf" along normal up to surface (89.5 mm away) from surface at 134.25 contours L4 A17 L17 | L4 A18 L15 | L4 A4 A7 A17 | L4 A17 L16 | L4 A9 A18 | L4 A18 L14 | L4 A4 A7 | L4 A9 | A13 | A14 picked at (31.228, 4.8338) picked at (65.228, 4.8338) picked at (32.7196, 6.7212) picked at (66.7196, 6.7212) bodies 8
extrude "Extrude50" add sketch "ReaderBodyHalf" along normal blind 5 from surface at 134.25 contours L4 A17 L17 | L4 A18 L15 | L4 A4 A7 A17 | L4 A17 L16 | L4 A9 A18 | L4 A18 L14 | L4 A4 A7 | L4 A9 picked at (31.228, 4.8338) picked at (65.228, 4.8338) picked at (32.7196, 6.7212) picked at (66.7196, 6.7212) bodies 8
extrude "Extrude52" add sketch "RelayBoxCrossSection" against normal blind 4 from surface at -7 contours L6 L21 L22 L24 | L6 L19 L22 L24 | L19 L22 L23 L24 bodies 8
extrude "Extrude51" cut sketch "RelayBoxCrossSection" against normal blind 7 contours A9 | A10 bodies 8
revolve "Revolve11" add 1 faces at (54, 8.3333, 136) angle 90 about axis through (61, 7, 136) along (1, 0, 0) on bodies 8 bodies 8
sketch "CarageBoltHoles" plane through (0, 0, 0) normal (0, -1, 0) x (1, 0, 0)
  circle A0 centre (18.5001, 30.5) radius 2.5
  circle A1 centre (82.5001, 56) radius 2.5
  circle A2 centre (82.5001, 5) radius 2.5
  line L0 (0, 0) -> (102, 0)
  line L1 (102, 0) -> (102, 134)
  line L2 (102, 134) -> (0, 134)
  line L3 (0, 134) -> (0, 0)
  line L4 (56.15, 46.7) -> (62.85, 46.7)
  line L5 (62.85, 46.7) -> (62.85, 40)
  line L6 (62.85, 40) -> (56.15, 40)
  line L7 (56.15, 40) -> (56.15, 46.7)
  line L8 (39.15, 46.7) -> (45.85, 46.7)
  line L9 (45.85, 40) -> (39.15, 40)
  line L10 (45.85, 46.7) -> (45.85, 40)
  line L11 (39.15, 40) -> (39.15, 46.7)
  line L12 (62.75, 89) -> (56.05, 89)
  line L13 (45.75, 89) -> (39.05, 89)
  line L14 (56.05, 95.7) -> (62.75, 95.7)
  line L15 (39.05, 95.7) -> (45.75, 95.7)
  line L16 (62.75, 95.7) -> (62.75, 89)
  line L17 (39.05, 89) -> (39.05, 95.7)
  line L18 (56.05, 89) -> (56.05, 95.7)
  line L19 (45.75, 95.7) -> (45.75, 89)
  circle A3 centre (18.5001, 30.5) radius 2.5
  circle A4 centre (82.5001, 56) radius 2.5
  circle A5 centre (82.5001, 5) radius 2.5
  line L20 (0, 0) -> (102, 0)
  line L21 (102, 0) -> (102, 134)
  line L22 (102, 134) -> (0, 134)
  line L23 (0, 134) -> (0, 0)
  circle A6 centre (59.4, 92.35) radius 10
  circle A7 centre (42.5, 92.35) radius 10
  point P0 (42.5, 92.35)
  point P1 (59.4, 92.35)
  dimension "d525" = 40
  dimension "d533" = 6.7
  dimension "d534" = 6.7
  dimension "d535" = 6.7
  dimension "d536" = 6.7
  dimension "d537" = 6.7
  dimension "d538" = 6.7
  dimension "d539" = 6.7
  dimension "d540" = 6.7
  dimension "d541" = 42.3
  dimension "d542" = 10.3
  dimension "d543" = 10.3
  dimension "d544" = 40
  dimension "d545" = 42.3
  dimension "d547" = 39.15
  dimension "d549" = 20
  dimension "d550" = 20
  constraint horizontal L4
  constraint vertical L5
  constraint horizontal L6
  constraint vertical L7
  constraint horizontal L8
  constraint vertical L10
  constraint horizontal L9
  constraint vertical L11
  constraint horizontal L14
  constraint vertical L16
  constraint horizontal L12
  constraint vertical L18
  constraint horizontal L15
  constraint vertical L19
  constraint horizontal L13
  constraint vertical L17
  constraint coincident P1 A6.centre
  constraint coincident P0 A7.centre
  measures "d525" distance of L0 L6
  measures "d533" distance of L17 L19
  measures "d534" distance of L13 L15
  measures "d535" distance of L12 L14
  measures "d536" distance of L16 L18
  measures "d537" distance of L4 L6
  measures "d538" distance of L5 L7
  measures "d539" distance of L8 L9
  measures "d540" distance of L10 L11
  measures "d541" distance of L4 L12
  measures "d542" distance of L7 L10
  measures "d543" distance of L18 L19
  measures "d544" distance of L0 L9
  measures "d545" distance of L8 L13
  measures "d547" distance of L3 L11
  measures "d549" diameter of A6
  measures "d550" diameter of A7
extrude "Extrude54" cut sketch "CarageBoltHoles" against normal blind 14 contours L4 L5 L6 L7 | L8 L9 L10 L11 | L12 L14 L16 L18 | L13 L15 L17 L19 bodies 1
extrude "Extrude55" add sketch "CarageBoltHoles" along normal blind 2 separate body contours A6 A7 | A6 A7 | A6 A7 makes body 9
move_body "Move5" bodies 9 to x (1, 0, 0) y (0, 1, 0) z (0, 0, 1) at (0, -25, 0)
equation "d1 = BoxLength"
equation "BoxLength = 102 mm"
equation "BoxWidth = 77 mm"
equation "CornerRadius = 4.5 mm"
equation "ReaderMountOffset = 11.5 mm"
equation "BoxHeight = 134 mm"
equation "InnerWidthL = 10 mm"
equation "d9 = InnerWidthW"
equation "d10 = InnerWidthW"
equation "M3HoleDiameter = 3.5 mm"
equation "ReaderMountPadding = 8 mm"
equation "d21 = M3HoleDiameter + ReaderMountPadding"
equation "d23 = M3HoleDiameter + ReaderMountPadding"
equation "d24 = M3HoleDiameter"
equation "d25 = M3HoleDiameter"
equation "d29 = ReaderMountOffset"
equation "d30 = ReaderMountOffset"
equation "d31 = ReaderMountOffset"
equation "d32 = ReaderMountOffset"
equation "d33 = ReaderMountOffset"
equation "d34 = ReaderMountOffset"
equation "d35 = ReaderMountOffset"
equation "d36 = ReaderMountOffset"
equation "d39 = BoxHeight"
equation "ReaderMountHeight = 6 mm"
equation "d44 = ReaderMountHeight"
equation "InnerWidthW = 7 mm"
equation "LidGap = 0.3 mm"
equation "M3HeadDiameter = 4.5 mm"
equation "M3InsertDiameter = 4.7 mm"
equation "M3InsertDepth = 4 mm"
equation "M3InsertOverhangDiameter = 10 mm"
equation "PingulpSrewDiameter = 5 mm"
equation "PingulpScrewHeadDiameter = 8.5 mm"
equation "PingulpScrewDepth = 4.75 mm"
equation "d138 = InnerWidthL"
equation "d166 = M3InsertDiameter"
equation "d167 = M3InsertOverhangDiameter"
equation "d168 = BoxLength / 3"
equation "d169 = M3InsertDiameter"
equation "d170 = M3InsertOverhangDiameter"
equation "d175 = M3InsertOverhangDiameter"
equation "d176 = M3InsertDiameter"
equation "d178 = BoxLength / 3"
equation "d179 = BoxLength / 3"
equation "d184 = M3InsertDiameter"
equation "d185 = M3InsertOverhangDiameter"
equation "d188 = M3InsertDepth * -2"
equation "d195 = M3InsertDepth * -1"
equation "d213 = M3InsertDepth * -2"
equation "d216 = M3InsertDepth * -1"
equation "d218 = M3InsertOverhangDiameter"
equation "d219 = M3InsertOverhangDiameter / 2"
equation "d221 = M3InsertDiameter"
equation "d222 = M3InsertDiameter"
equation "d223 = M3InsertDiameter"
equation "d224 = M3InsertDiameter"
equation "d225 = M3InsertOverhangDiameter"
equation "d226 = M3InsertOverhangDiameter"
equation "d227 = M3InsertOverhangDiameter"
equation "d231 = M3InsertOverhangDiameter / 2"
equation "d232 = M3InsertOverhangDiameter / 2"
equation "d233 = M3InsertOverhangDiameter / 2"
equation "d237 = BoxWidth"
equation "LcdLength = 51 mm"
equation "LcdWidth = 20 mm"
equation "d244 = LcdLength"
equation "d245 = LcdWidth"
equation "d246 = ( BoxWidth - LcdLength ) / 2"
equation "d248 = LcdDepth * -1"
equation "LcdBoardWidth = 27 mm"
equation "LcdDepth = 8 mm"
equation "d252 = LcdLength"
equation "d253 = LcdBoardWidth"
equation "d254 = ( LcdBoardWidth - LcdWidth ) / 2"
equation "d255 = ( BoxWidth - LcdLength ) / 2"
equation "d256 = LcdDepth * -1"
equation "LcdMountHoleSpacingL = 43.5 mm"
equation "LcdMountHoleSpacingW = 23 mm"
equation "M2SelfTapDiameter = 2 mm"
equation "M2SelfTapDepth = 4 mm"
equation "d262 = M2SelfTapDiameter"
equation "d263 = ( LcdLength - LcdMountHoleSpacingL ) / 2"
equation "d264 = ( LcdBoardWidth - LcdMountHoleSpacingW ) / 2"
equation "d265 = M2SelfTapDiameter"
equation "d266 = M2SelfTapDiameter"
equation "d267 = M2SelfTapDiameter"
equation "d268 = LcdMountHoleSpacingL"
equation "d269 = LcdMountHoleSpacingW"
equation "d270 = LcdMountHoleSpacingL"
equation "d271 = LcdMountHoleSpacingW"
equation "d272 = ( LcdBoardWidth - LcdMountHoleSpacingW ) / 2"
equation "d274 = M2SelfTapDepth"
equation "d282 = ( BoxWidth - 51 mm ) / 2"
equation "d284 = M3InsertDiameter"
equation "d285 = M3InsertDiameter"
equation "d290 = M3InsertOverhangDiameter"
equation "d291 = M3InsertOverhangDiameter"
equation "d293 = M3InsertDepth * -1"
equation "d295 = M3HoleDiameter"
equation "d296 = M3HoleDiameter"
equation "d297 = M3HoleDiameter"
equation "d298 = M3HoleDiameter"
equation "d303 = BoxWidth / 3"
equation "d327 = PingulpSrewDiameter"
equation "d328 = PingulpSrewDiameter"
equation "d329 = PingulpSrewDiameter"
equation "d334 = 11 mm + ( 51 / 2 ) * 1 mm"
equation "d335 = 6.5 mm + 64 mm"
equation "d336 = PingulpScrewHeadDiameter"
equation "d337 = PingulpScrewHeadDiameter"
equation "d338 = PingulpScrewHeadDiameter"
equation "d340 = BoxWidth / 2"
equation "d345 = CornerRadius"
equation "d346 = M3InsertDiameter"
equation "d347 = M3InsertDiameter"
equation "d349 = M3InsertOverhangDiameter"
equation "d350 = M3InsertOverhangDiameter"
equation "d366 = CornerRadius"
equation "d384 = BoxHeight"
equation "d392 = M3HoleDiameter"
equation "d393 = M3HoleDiameter"
equation "d394 = M3HoleDiameter"
equation "d398 = CornerRadius"
equation "d419 = M3InsertDiameter"
equation "d420 = M3InsertDiameter"
equation "d421 = M3InsertDiameter"
equation "d422 = M3InsertDiameter"
equation "d425 = M3InsertDiameter * 2"
equation "d426 = M3InsertDiameter * 2"
equation "d427 = M3InsertDiameter * 2"
equation "d428 = M3InsertDiameter * 2"
equation "d431 = -M3InsertDepth"
equation "RelayBoxDepth = 94 mm"
equation "d435 = RelayBoxDepth"
equation "d452 = M3InsertDiameter"
equation "d453 = M3InsertDiameter"
equation "d454 = M3InsertDiameter"
equation "d455 = M3InsertDiameter"
equation "d456 = M3InsertDiameter * 2"
equation "d457 = M3InsertDiameter * 2"
equation "d458 = M3InsertDiameter * 2"
equation "d459 = M3InsertDiameter * 2"
equation "d463 = M3InsertDepth"
equation "M3ScrewHeadDiameter = 6 mm"
equation "d470 = M3ScrewHeadDiameter"
equation "d471 = M3ScrewHeadDiameter"
equation "d472 = M3ScrewHeadDiameter"
equation "d494 = M3InsertDiameter"
equation "d495 = M3InsertDiameter * 2"
equation "d496 = 26.5 mm + ( 49.4 / 2 ) * 1 mm"
equation "d498 = -M3InsertDepth"
equation "RelayBoxLidMargin = 0.25 mm"
equation "d515 = RelayBoxLidMargin"
equation "d516 = RelayBoxLidMargin"